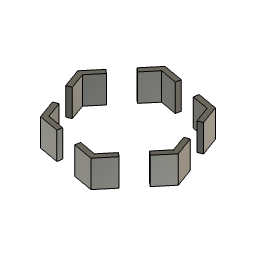
ServoBase v2 (Autodesk Fusion 360 design; units mm, degrees)
Autodesk Fusion 360 part; units mm, degrees
sketch "Sketch1" plane through (0, 0, 0) normal (0, 0, 1) x (1, 0, 0)
  line L0 (-10.798, 13.3938) -> (-13.526, 20.8958)
  line L1 (-9.4934, 25.6987) -> (-13.526, 20.8958)
  line L2 (19.2845, 47.1681) -> (9.9209, 48.822)
  line L3 (55.6112, 15.5789) -> (58.2905, 8.2107)
  line L4 (52.0708, 0.8027) -> (58.2905, 8.2107)
  line L5 (8.3931, -15.0435) -> (-1.0646, -13.373)
  line L6 (23.8122, -14.7206) -> (23.2904, -17.6748)
  line L7 (10.4886, -15.4136) -> (11.0104, -12.4594)
  line L8 (48.4491, 1.1547) -> (50.7467, -0.7743)
  line L9 (42.3875, -10.7304) -> (40.0899, -8.8014)
  line L10 (47.0192, 30.4285) -> (49.8385, 31.4537)
  line L11 (54.2812, 19.2364) -> (51.4618, 18.2112)
  line L12 (20.9523, 43.827) -> (21.4741, 46.7813)
  line L13 (34.276, 44.5201) -> (33.7542, 41.5658)
  line L14 (-3.6845, 27.9518) -> (-5.9821, 29.8808)
  line L15 (2.3771, 39.8369) -> (4.6746, 37.9079)
  line L16 (-2.2546, -1.322) -> (-5.074, -2.3473)
  line L17 (-9.5166, 9.87) -> (-6.6972, 10.8953)
  line L18 (-10.798, 13.3938) -> (-9.5166, 9.87)
  line L19 (-5.074, -2.3473) -> (-1.0646, -13.373)
  line L20 (1.1628, -10.72) -> (-2.2546, -1.322)
  line L21 (-6.6972, 10.8953) -> (-10.1147, 20.2932)
  line L22 (33.6598, -16.4599) -> (23.8122, -14.7206)
  line L23 (11.0104, -12.4594) -> (1.1628, -10.72)
  line L24 (8.3931, -15.0435) -> (10.4886, -15.4136)
  line L25 (23.2904, -17.6748) -> (34.8436, -19.7155)
  line L26 (54.8793, 8.8133) -> (48.4491, 1.1547)
  line L27 (40.0899, -8.8014) -> (33.6598, -16.4599)
  line L28 (52.0708, 0.8027) -> (50.7467, -0.7743)
  line L29 (42.3875, -10.7304) -> (34.8436, -19.7155)
  line L30 (43.6017, 39.8265) -> (47.0192, 30.4285)
  line L31 (51.4618, 18.2112) -> (54.8793, 8.8133)
  line L32 (55.6112, 15.5789) -> (54.2812, 19.2364)
  line L33 (49.8385, 31.4537) -> (45.8292, 42.4795)
  line L34 (11.1048, 45.5664) -> (20.9523, 43.827)
  line L35 (33.7542, 41.5658) -> (43.6017, 39.8265)
  line L36 (19.2845, 47.1681) -> (21.4741, 46.7813)
  line L37 (34.276, 44.5201) -> (45.8292, 42.4795)
  line L38 (-10.1147, 20.2932) -> (-3.6845, 27.9518)
  line L39 (4.6746, 37.9079) -> (11.1048, 45.5664)
  line L40 (-9.4934, 25.6987) -> (-5.9821, 29.8808)
  line L41 (2.3771, 39.8369) -> (9.9209, 48.822)
  constraint parallel L6 L7
  constraint parallel L8 L9
  constraint parallel L10 L11
  constraint parallel L12 L13
  constraint parallel L14 L15
  constraint parallel L16 L17
  constraint coincident L16.end L18
  constraint collinear L18 L19
  constraint collinear L20 L21
  constraint coincident L13.start L36
  constraint coincident L15.start L40
  constraint coincident L6.end L24
  constraint coincident L9.start L28
  constraint coincident L10.end L32
  constraint collinear L22 L23
  constraint collinear L24 L25
  constraint collinear L26 L27
  constraint collinear L28 L29
  constraint collinear L30 L31
  constraint collinear L32 L33
  constraint collinear L34 L35
  constraint collinear L36 L37
  constraint collinear L38 L39
  constraint collinear L40 L41
extrude "Extrude1" add sketch "Sketch1" along normal blind 16 makes body 1 at (-8.4967, 26.8858, 5.3333) makes body 2 at (55.6177, 15.5612, 5.3333) makes body 3 at (4.8917, 42.8319, 5.3333) makes body 4 at (6.6375, -14.7334, 5.3333) makes body 5 at (39.8729, -13.7254, 5.3333) makes body 6 at (38.1271, 43.8399, 5.3333)
